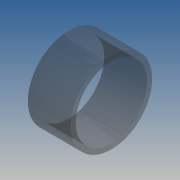
# Autodesk Inventor part: P22
Saved by Autodesk Inventor 2012 SP1 (Build 160190100, 190)
## iProperties
Created: 2012-07-17
Part Number: P22
Material: PC (Transp. / Durchsicht.)
Description: Protection réducteur
Document SubType Name: Modeling
Designer: sta
Mass: 7.42201 g
Surface Area: 55.3706 cm^2
Volume: 6.18501 cm^3
Density: 1.2 g/cm^3
Title: Kart 2012
Author: sta
Autodesk Inventor part; units mm, degrees
ref_plane "YZ Plane" through (0, 0, 0) normal (1, 0, 0) x (0, 1, 0)
ref_plane "XZ Plane" through (0, 0, 0) normal (0, 1, 0) x (-1, 0, 0)
ref_plane "XY Plane" through (0, 0, 0) normal (0, 0, 1) x (1, 0, 0)
sketch "Sketch1" plane through (0, 0, 0) normal (0, 0, 1) x (1, 0, 0)
  line L0 (0, 0) -> (23.5766, 0)
  line L1 (0, 0) -> (0, 20)
  line L2 (0, 20) -> (21, 20)
  line L3 (21, 20) -> (21, 0)
  line L4 (0, 17.5) -> (21, 17.5)
  dimension "d0" = 40
  dimension "d1" = 21
  dimension "d2" = 35
  constraints: 10 end point, 4 perpendicular, 3 point on line, 1 horizontal
  measures "d0" diameter of L2 L0
  measures "d1" distance of L1.end L2.end
  measures "d2" diameter of L4 L0
revolve "Revolution1" add sketch "Sketch1" angle 360 about axis through (0, 0, 0) along (1, 0, 0) contours L1 L2 L3 L4
body "Solid1"
